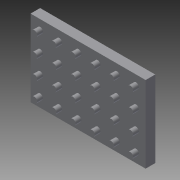
# Autodesk Inventor part: p
Saved by Autodesk Inventor 2015 (Build 190159000, 159)
## iProperties
Created: 2015-02-06
Part Number: p
Material: Generic
Document SubType Name: Modeling
Designer: PLTW-Stu-02
Density: 1 g/cm^3
Appearance: Default
Author: PLTW-Stu-02
Autodesk Inventor part; units mm, degrees
ref_plane "YZ Plane" through (0, 0, 0) normal (1, 0, 0) x (0, 1, 0)
ref_plane "XZ Plane" through (0, 0, 0) normal (0, 1, 0) x (-1, 0, 0)
ref_plane "XY Plane" through (0, 0, 0) normal (0, 0, 1) x (1, 0, 0)
sketch "Sketch1" plane through (0, 0, 0) normal (0, 0, 1) x (1, 0, 0)
  line L0 (12.4728, 9.7682) -> (164.8728, 9.7682)
  line L1 (164.8728, 9.7682) -> (164.8728, 111.3682)
  line L2 (164.8728, 111.3682) -> (12.4728, 111.3682)
  line L3 (12.4728, 111.3682) -> (12.4728, 9.7682)
  point P0 (0, 0)
  dimension "d0" = 152.4
  dimension "d1" = 101.6
  constraints: 8 end point, 2 parallel, 1 horizontal, 1 perpendicular
  measures "d0" distance of L2.end L1.end
  measures "d1" distance of L1.end L0.end
extrude "Extrusion1" add sketch "Sketch1" along normal blind 12.7
sketch "Sketch2" plane through (0, 0, 12.7) normal (0, 0, 1) x (1, 0, 0)
  circle A0 centre (25.1728, 22.4682) radius 3.81
  line L0 (12.4728, 111.3682) -> (12.4728, 9.7682) projected
  line L1 (12.4728, 9.7682) -> (164.8728, 9.7682) projected
  circle A1 centre (25.1728, 47.8682) radius 3.81
  circle A2 centre (25.1728, 73.2682) radius 3.81
  circle A3 centre (25.1728, 98.6682) radius 3.81
  circle A4 centre (50.5728, 22.4682) radius 3.81
  circle A5 centre (50.5728, 47.8682) radius 3.81
  circle A6 centre (50.5728, 73.2682) radius 3.81
  circle A7 centre (50.5728, 98.6682) radius 3.81
  circle A8 centre (75.9728, 22.4682) radius 3.81
  circle A9 centre (75.9728, 47.8682) radius 3.81
  circle A10 centre (75.9728, 73.2682) radius 3.81
  circle A11 centre (75.9728, 98.6682) radius 3.81
  circle A12 centre (101.3728, 22.4682) radius 3.81
  circle A13 centre (101.3728, 47.8682) radius 3.81
  circle A14 centre (101.3728, 73.2682) radius 3.81
  circle A15 centre (101.3728, 98.6682) radius 3.81
  circle A16 centre (126.7728, 22.4682) radius 3.81
  circle A17 centre (126.7728, 47.8682) radius 3.81
  circle A18 centre (126.7728, 73.2682) radius 3.81
  circle A19 centre (126.7728, 98.6682) radius 3.81
  circle A20 centre (152.1728, 22.4682) radius 3.81
  circle A21 centre (152.1728, 47.8682) radius 3.81
  circle A22 centre (152.1728, 73.2682) radius 3.81
  circle A23 centre (152.1728, 98.6682) radius 3.81
  point P0 (0, 0)
  dimension "d4" = 7.62
  dimension "d5" = 12.7
  dimension "d6" = 12.7
  dimension "d9" = 25.4
  dimension "d12" = 25.4
  constraints: 24 centre point, 1 horizontal, 1 vertical, 46 other
  measures "d4" diameter of A0
  measures "d5" distance from line of L0 A0.centre
  measures "d6" distance from line of L1 A0.centre
  measures "d9" distance of A0.centre A1.centre
  measures "d12" distance of A0.centre A4.centre
extrude "Extrusion2" add sketch "Sketch2" along normal blind 7.62
body "Solid1"
